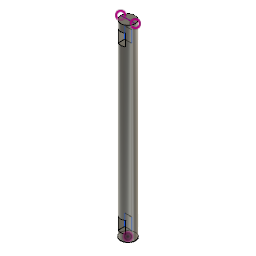
Arm Wheel Dowel Pin (Autodesk Fusion 360 design; units mm, degrees)
Autodesk Fusion 360 part; units mm, degrees
sketch "Sketch1" plane through (0, 0, 0) normal (0, 0, 1) x (1, 0, 0)
  circle A0 centre (0, 0) radius 3.1
  dimension "d3" = 6.2
  constraint coincident A0.centre origin
  measures "d3" diameter of A0
extrude "Extrude1" add sketch "Sketch1" along normal blind 80
sketch "Sketch3" plane through (0, 0, 0) normal (0, 1, 0) x (1, 0, 0)
  line L0 (-1.4286, -3) -> (1.5714, -3)
  line L1 (1.5714, -3) -> (1.5714, -8)
  line L2 (1.5714, -8) -> (-1.4286, -8)
  line L3 (-1.4286, -8) -> (-1.4286, -3)
  line L4 (-1.4286, -77) -> (1.5714, -77)
  line L5 (1.5714, -77) -> (1.5714, -72)
  line L6 (1.5714, -72) -> (-1.4286, -72)
  line L7 (-1.4286, -72) -> (-1.4286, -77)
  line L8 (-3.1, -80) -> (3.1, -80)
  dimension "d9" = 3
  dimension "d10" = 5
  dimension "d11" = 3
  dimension "d12" = 5
  dimension "d18" = 3
  dimension "d19" = 3
  constraint horizontal L0
  constraint vertical L1
  constraint horizontal L2
  constraint vertical L3
  constraint horizontal L4
  constraint vertical L5
  constraint horizontal L6
  constraint vertical L7
  measures "d9" distance of L0.start L0.end
  measures "d10" distance of L0.start L2.end
  measures "d11" distance of L4.start L4.end
  measures "d12" distance of L4.start L6.end
  measures "d18" distance of L0 origin
  measures "d19" distance of L4 L8
extrude "Extrude2" cut sketch "Sketch3" along normal mid plane 200 contours L4 L5 L6 L7
extrude "Extrude3" cut sketch "Sketch3" along normal mid plane 200 contours L0 L1 L2 L3
equation "dowel_pin_radius = 3.10 mm"
equation "length = 80 mm"
equation "d3 = dowel_pin_radius * 2"
equation "d4 = length"
equation "hole_distance = 3 mm"
equation "hole_width = 3 mm"
equation "hole_height = 5 mm"
equation "d9 = hole_width"
equation "d10 = hole_height"
equation "d11 = hole_width"
equation "d12 = hole_height"
equation "extra = 100 mm"
equation "d14 = extra"
equation "d16 = extra"
equation "d18 = hole_distance"
equation "d19 = hole_distance"
